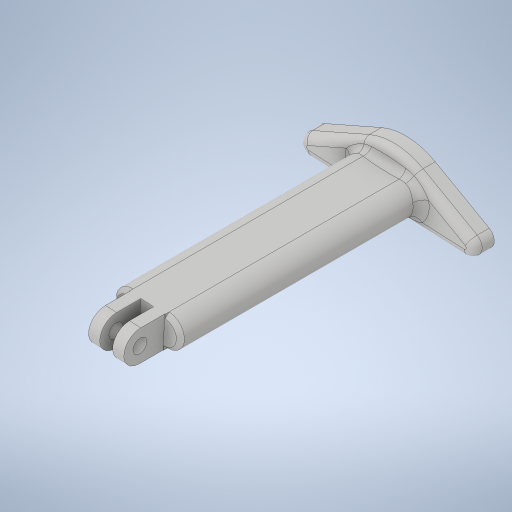
# Autodesk Inventor part: Camera stand
Saved by Autodesk Inventor 2024 (Build 280153000, 153)
## iProperties
Created: 2019-06-22
Part Number: Camera stand
Material: Generic
Document SubType Name: Modeling
Designer: infinity
Density: 1 g/cm^3
Appearance: Default
Author: infinity
Autodesk Inventor part; units mm, degrees
note: some values were not read from the file. Chosen so that the rebuilt part matches the saved one: direction of "Hole2".
ref_plane "YZ Plane" through (0, 0, 0) normal (1, 0, 0) x (0, 1, 0)
ref_plane "XZ Plane" through (0, 0, 0) normal (0, 1, 0) x (-1, 0, 0)
ref_plane "Work Plane1" through (-6.8158, 0.172, 0) normal (0, 0, 1) x (0.9987277, -0.0504278, 0)
sketch "Sketch1" plane through (-6.8158, 0.172, 0) normal (0, 0, 1) x (0.9987277, -0.0504278, 0)
  circle A0 centre (0, 135.16) radius 1.5 projected
  line L0 (19.4098, 129.16) -> (-19.4098, 129.16)
  line L1 (-20.5279, 133.8961) -> (-6.7082, 140.8059)
  line L2 (6.7082, 140.8059) -> (20.5279, 133.8961)
  arc A1 (19.4098, 129.16) -> (20.5279, 133.8961) centre (19.4098, 131.66) ccw
  arc A2 (-20.5279, 133.8961) -> (-19.4098, 129.16) centre (-19.4098, 131.66) ccw
  arc A3 (6.7082, 140.8059) -> (-6.7082, 140.8059) centre (0, 127.3895) ccw
  point P0 (6.8158, 0.172)
  point P1 (30, 129.16)
  point P2 (-30, 129.16)
  point P3 (0, 144.16)
  dimension "d0" = 0
  dimension "d1" = 60
  dimension "d2" = 15
  dimension "d3" = 30
  dimension "d4" = 6
  dimension "d5" = 2.5
  dimension "d6" = 15
  constraints: 6 end point, 6 point on circle, 6 point on line, 6 tangent, 3 centre point, 1 equal radius, 1 horizontal
  measures "d0" horizontal distance of A0.centre point (0, 144.16)
  measures "d1" distance of point (30, 129.16) point (-30, 129.16)
  measures "d2" distance from line of point (0, 144.16) L0
  measures "d3" horizontal distance of point (30, 129.16) A0.centre
  measures "d4" distance from line of L0 A0.centre
  measures "d5" radius of A1
  measures "d6" radius of A3
extrude "Extrusion1" add sketch "Sketch1" along normal blind 5 contours A0 | L0 A2 L1 A3 L2 A1
sketch "Sketch2" plane through (-6.8158, 0.172, 0) normal (0, 0, -1) x (-0.9987277, 0.0504278, 0)
  circle A0 centre (16.5006, 132.1631) radius 1.5 projected
  circle A1 centre (0, 135.16) radius 1.5 projected
  circle A2 centre (-16.4994, 132.1569) radius 1.5 projected
  point P0 (-6.8158, 0.172)
  constraints: 3 coincident
hole "Hole1" at (16.327, 131.3287, 0) at (-16.6307, 132.999, 0) direction (0, 0, 1) diameter 2.8 depth 4.5
fillet "Fillet1" radius 2 6 edges at (-13.4902, 138.0349, 5) (-22.0206, 132.1923, 5) (-0.3026, 129.1676, 5) (21.6097, 129.9893, 5) (13.7112, 136.6615, 5) (0.3646, 142.3803, 5)
sketch "Sketch3" plane through (-6.8158, 0.172, 5) normal (0, 0, 1) x (0.9987277, -0.0504278, 0)
  circle A0 centre (0, 135.16) radius 1.5 projected
  line L0 (4.5, 135.16) -> (-4.5, 135.16) construction
  line L1 (4.5, 139.16) -> (-4.5, 139.16)
  line L2 (-4.5, 131.16) -> (4.5, 131.16)
  arc A1 (4.5, 131.16) -> (4.5, 139.16) centre (4.5, 135.16) ccw
  arc A2 (-4.5, 139.16) -> (-4.5, 131.16) centre (-4.5, 135.16) ccw
  point P0 (6.8158, 0.172)
  dimension "d19" = 0
  dimension "d23" = 0
  dimension "d24" = 8
  dimension "d25" = 9
  constraints: 8 end point, 4 point on circle, 4 tangent, 2 centre point, 1 horizontal, 1 midpoint, 1 parallel
  measures "d19" distance of A0.centre point (0, 135.16)
  measures "d23" distance of A0.centre point (0, 135.16)
  measures "d24" distance between parallel lines of L1 L2
  measures "d25" distance of L0.end L0.start
extrude "Extrusion2" add sketch "Sketch3" along normal blind 60 contours A0 | A1 L2 A2 L1
fillet "Fillet2" radius 2 4 edges at (8.4892, 134.7314, 5) (-0.2017, 131.1651, 5) (-8.4892, 135.5886, 5) (0.2017, 139.1549, 5)
sketch "Sketch4" plane through (-6.8158, 0.172, 65) normal (0, 0, 1) x (0.9987277, -0.0504278, 0)
  line L0 (4.5, 131.16) -> (-4.5, 131.16) projected
  line L1 (4.5, 139.16) -> (-4.5, 139.16) projected
  line L2 (-4.5, 131.16) -> (-1.5, 131.16)
  line L3 (-1.5, 131.16) -> (-1.5, 139.16)
  line L4 (-1.5, 139.16) -> (-4.5, 139.16)
  line L5 (-4.5, 139.16) -> (-4.5, 131.16)
  line L6 (4.5, 131.16) -> (1.5, 131.16)
  line L7 (1.5, 131.16) -> (1.5, 139.16)
  line L8 (1.5, 139.16) -> (4.5, 139.16)
  line L9 (4.5, 139.16) -> (4.5, 131.16)
  point P0 (6.8158, 0.172)
  dimension "d27" = 3
  dimension "d28" = 3
  dimension "d29" = 3
  constraints: 16 end point, 4 parallel, 3 point on line, 2 horizontal, 2 perpendicular
  measures "d27" distance between parallel lines of L7 L3
  measures "d28" distance from line of L7 L8.end
  measures "d29" distance between parallel lines of L5 L3
extrude "Extrusion3" add sketch "Sketch4" along normal blind 10 contours L0 L7 L1 L9 | L0 L5 L1 L3
fillet "Fillet3" radius 4 4 edges at (-3.1979, 131.3164, 75) (2.7945, 131.0138, 75) (3.1979, 139.0036, 75) (-2.7945, 139.3062, 75)
chamfer "Chamfer1" distance 1 angle 45 2 edges at (-8.4892, 135.5886, 65) (8.4892, 134.7314, 65)
sketch "Sketch5" plane through (4.3934, 132.9356, 45) normal (0.9987277, -0.0504278, 0) x (0, 0, -1)
  line L0 (0, 0) -> (0, 4) projected
  line L1 (-19, 6) -> (-26, 6) projected
  point P0 (45, -132.988)
  point P1 (-26, 2)
  dimension "d37" = 4
  dimension "d59" = 0
  measures "d37" distance from line of point (-26, 2) L1
  measures "d59" horizontal distance of point (-26, 2) L1.end
hole "Hole2" at (4.4943, 134.9331, 71) direction (-0.9987277, 0.0504278, 0) diameter 3.5 depth 9
sketch "Sketch6" plane through (-6.8158, 0.172, 0) normal (0, 0, -1) x (-0.9987277, 0.0504278, 0)
  circle A0 centre (0, 135.16) radius 1.5 projected
  point P0 (-6.8158, 0.172)
  constraints: 1 coincident
hole "Hole3" at (0, 135.16, 0) direction (0, 0, 1) diameter 2.8 depth 7
sketch "Sketch7" plane through (-6.8158, 0.172, 65) normal (0, 0, 1) x (0.9987277, -0.0504278, 0)
  line L0 (-1.6, 113.5463) -> (1.6, 113.5463)
  line L1 (1.6, 113.5463) -> (1.6, 145.903)
  line L2 (1.6, 145.903) -> (-1.6, 145.903)
  line L3 (-1.6, 145.903) -> (-1.6, 113.5463)
  line L4 (-5.6829, 111.8123) -> (-4.4, 111.8123)
  line L5 (-4.4, 111.8123) -> (-4.4, 142.6037)
  line L6 (-4.4, 142.6037) -> (-5.6829, 142.6037)
  line L7 (-5.6829, 142.6037) -> (-5.6829, 111.8123)
  line L8 (10.3251, 112.1591) -> (4.4, 112.1591)
  line L9 (4.4, 112.1591) -> (4.4, 145.9114)
  line L10 (4.4, 145.9114) -> (10.3251, 145.9114)
  line L11 (10.3251, 145.9114) -> (10.3251, 112.1591)
  circle A0 centre (0, 135.16) radius 1.4 projected
  line L12 (-4.5, 131.16) -> (-4.5, 139.16) projected
  line L13 (4.5, 139.16) -> (4.5, 131.16) projected
  point P0 (6.8158, 0.172)
  dimension "d52" = 3.2
  dimension "d53" = 1.6
  dimension "d54" = 0.1
  dimension "d55" = 0.1
  constraints: 24 end point, 6 parallel, 3 horizontal, 3 perpendicular
  measures "d52" distance between parallel lines of L1 L3
  measures "d53" distance from line of A0.centre L3
  measures "d54" distance between parallel lines of L12 L5
  measures "d55" distance between parallel lines of L13 L9
extrude "Extrusion4" cut sketch "Sketch7" along normal through all
equation "\"d3\" = 0.5 * d1"
equation "\"d53\" = 0.5 * d52"
equation "\"d55\" = d54"
body "Solid1"
